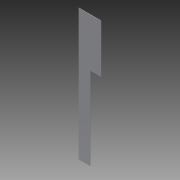
# Autodesk Inventor part: Fa
Saved by Autodesk Inventor 2014 SP1 (Build 180222100, 222)
## iProperties
Created: 2015-03-28
Part Number: Fa
Material: LCP Plastic
Document SubType Name: Modeling
Designer: tuleu
Density: 1.626 g/cm^3
Appearance: PVC - White
Author: tuleu
Autodesk Inventor part; units mm, degrees
ref_plane "YZ Plane" through (0, 0, 0) normal (1, 0, 0) x (0, 1, 0)
ref_plane "XZ Plane" through (0, 0, 0) normal (0, 1, 0) x (-1, 0, 0)
ref_plane "XY Plane" through (0, 0, 0) normal (0, 0, 1) x (1, 0, 0)
sketch "Sketch1" plane through (0, 0, 0) normal (0, 1, 0) x (-1, 0, 0)
  line L0 (90, -525) -> (-5, -525)
  line L1 (-90, 135) -> (-90, 525)
  line L2 (-90, 525) -> (90, 525)
  line L3 (90, 525) -> (90, -525)
  line L4 (-5, -525) -> (-5, 135)
  line L5 (-5, 135) -> (-90, 135)
  line L6 (0, 525) -> (0, -525)
  line L7 (90, 0) -> (-5, 0)
  point P0 (0, 0)
  dimension "d0" = 180
  dimension "d1" = 1050
  dimension "d2" = 660
  dimension "d3" = 95
  constraints: 16 end point, 4 perpendicular, 3 midpoint, 3 parallel, 3 point on line, 1 horizontal
  measures "d0" distance between parallel lines of L1 L3
  measures "d1" distance of L2.end L0.start
  measures "d2" distance of L0.end L4.end
  measures "d3" distance of L0.start L0.end
extrude "Extrusion1" add sketch "Sketch1" along normal blind 2
body "Solid1"
